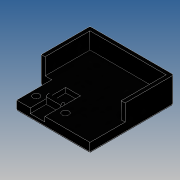
# Autodesk Inventor part: Tapa del cable
Saved by Autodesk Inventor 2016 (Build 200138000, 138)
## iProperties
Created: 2016-05-25
Part Number: Tapa del cable
Material: ABS Plastic
Document SubType Name: Modeling
Designer: Familia
Density: 1.06 g/cm^3
Appearance: Black
Mass: 10.4624 g
Surface Area: 60.6461 cm^2
Volume: 9.87015 cm^3
Author: Familia
Autodesk Inventor part; units mm, degrees
ref_plane "YZ Plane" through (0, 0, 0) normal (1, 0, 0) x (0, 1, 0)
ref_plane "XZ Plane" through (0, 0, 0) normal (0, 1, 0) x (-1, 0, 0)
ref_plane "XY Plane" through (0, 0, 0) normal (0, 0, 1) x (1, 0, 0)
sketch "Sketch1" plane through (0, 0, 0) normal (0, 0, 1) x (1, 0, 0)
  line L0 (-21.5, -21.5) -> (21.5, -21.5)
  line L1 (21.5, -21.5) -> (21.5, 21.5)
  line L2 (21.5, 21.5) -> (-21.5, 21.5)
  line L3 (-21.5, 21.5) -> (-21.5, -21.5)
  line L4 (-21.5, -21.5) -> (21.5, 21.5) construction
  line L5 (21.5, -21.5) -> (-21.5, 21.5) construction
  point P0 (0, 0)
  dimension "d0" = 43
  dimension "d1" = 43
  constraints: 12 end point, 2 midpoint, 2 parallel, 1 horizontal, 1 perpendicular
  measures "d0" distance of L1.end L2.end
  measures "d1" distance of L2.end L0.start
extrude "Extrusion1" add sketch "Sketch1" along normal blind 13.5
sketch "Sketch2" plane through (0, 0, 13.5) normal (0, 0, 1) x (1, 0, 0)
  line L0 (19.5, -19.5) -> (-19.5, -19.5)
  line L1 (-19.5, -19.5) -> (-19.5, 19.5)
  line L2 (-19.5, 19.5) -> (19.5, 19.5)
  line L3 (19.5, 19.5) -> (19.5, -19.5)
  line L4 (19.5, -19.5) -> (-19.5, 19.5) construction
  line L5 (-19.5, -19.5) -> (19.5, 19.5) construction
  line L6 (-21.5, 21.5) -> (-21.5, -21.5) construction
  line L7 (21.5, 21.5) -> (-21.5, 21.5) construction
  point P0 (0, 0)
  dimension "d4" = 2
  dimension "d5" = 2
  constraints: 12 end point, 2 midpoint, 2 parallel, 1 horizontal, 1 perpendicular
  measures "d4" distance between parallel lines of L2 L7
  measures "d5" distance between parallel lines of L6 L1
extrude "Extrusion2" cut sketch "Sketch2" against normal blind 8.5
sketch "Sketch3" plane through (0, 0, 13.5) normal (0, 0, 1) x (1, 0, 0)
  line L0 (-21.5, -3.5) -> (21.5, -3.5)
  line L1 (21.5, -3.5) -> (21.5, -28.5)
  line L2 (21.5, -28.5) -> (-21.5, -28.5)
  line L3 (-21.5, -28.5) -> (-21.5, -3.5)
  line L4 (-21.5, -21.5) -> (21.5, -21.5) projected
  line L5 (-21.5, 21.5) -> (-21.5, -21.5) projected
  line L6 (21.5, -21.5) -> (21.5, 21.5) projected
  point P0 (0, 0)
  dimension "d8" = 18
  dimension "d9" = 25
  constraints: 8 end point, 2 parallel, 2 point on line, 1 horizontal, 1 perpendicular
  measures "d8" distance between parallel lines of L4 L0
  measures "d9" distance between parallel lines of L2 L0
extrude "Extrusion3" cut sketch "Sketch3" against normal up to surface (8.5 mm away)
sketch "Sketch4" plane through (0, 0, 5) normal (0, 0, 1) x (1, 0, 0)
  line L0 (-21.5, -3.5) -> (-19.5, -3.5) projected
  line L1 (21.5, -21.5) -> (-21.5, -21.5) projected
  line L2 (-21.5, -3.5) -> (-16.1, -3.5)
  line L3 (-16.1, -3.5) -> (-16.1, -21.5)
  line L4 (-16.1, -21.5) -> (-21.5, -21.5)
  line L5 (-21.5, -21.5) -> (-21.5, -3.5)
  point P0 (0, 0)
  dimension "d12" = 5.4
  constraints: 8 end point, 2 parallel, 1 horizontal, 1 perpendicular, 1 point on line
  measures "d12" distance between parallel lines of L5 L3
extrude "Extrusion4" cut sketch "Sketch4" against normal through all
sketch "Sketch5" plane through (0, 0, 5) normal (0, 0, 1) x (1, 0, 0)
  line L0 (-9.1, -21.5) -> (-1.6, -21.5)
  line L1 (-1.6, -21.5) -> (-1.6, -3.3)
  line L2 (-1.6, -3.3) -> (-9.1, -3.3)
  line L3 (-9.1, -3.3) -> (-9.1, -21.5)
  line L4 (21.5, -21.5) -> (-16.1, -21.5) construction
  line L5 (-16.1, -3.5) -> (-16.1, -21.5) construction
  line L6 (-12.85, -14.7) -> (-9.1, -14.7) construction
  line L7 (-1.6, -14.7) -> (2.15, -14.7) construction
  point P0 (0, 0)
  dimension "d15" = 7
  dimension "d16" = 7.5
  dimension "d17" = 18.2
  dimension "d18" = 15
  dimension "d19" = 6.8
  constraints: 12 end point, 4 point on line, 2 horizontal, 2 parallel, 2 perpendicular, 1 collinear, 1 horizontal alignment
  measures "d15" distance between parallel lines of L3 L5
  measures "d16" distance of L1.end L2.end
  measures "d17" distance of L0.end L1.end
  measures "d18" distance of L7.end L6.start
  measures "d19" distance from line of L6.start L4
extrude "Extrusion5" cut sketch "Sketch5" against normal blind 2.5
sketch "Sketch6" plane through (0, 0, 2.5) normal (0, 0, 1) x (1, 0, 0)
  line L0 (-9.1, -11.5) -> (-1.6, -11.5)
  line L1 (-1.6, -11.5) -> (-1.6, -13.3)
  line L2 (-1.6, -13.3) -> (-9.1, -13.3)
  line L3 (-9.1, -13.3) -> (-9.1, -11.5)
  line L4 (-9.1, -21.5) -> (-9.1, -3.3) construction
  line L5 (-1.6, -3.3) -> (-1.6, -21.5) construction
  point P0 (0, 0)
  point P1 (-9.1, -12.4)
  dimension "d22" = 1.8
  constraints: 8 end point, 2 midpoint, 2 parallel, 2 point on line, 1 horizontal, 1 perpendicular
  measures "d22" distance between parallel lines of L2 L0
extrude "Extrusion6" add sketch "Sketch6" along normal blind 4.2
full round fillet "Fillet1" first side at (-4.1, -13.3, 3.3333) centre faces at (-6.6, -12.1, 6.7) second side at (-6.6, -11.5, 3.3333)
fillet "Fillet2" radius 0.8 6 edges at (21.5, 21.5, 6.75) (-21.5, 21.5, 6.75) (-21.5, 9, 0) (0, 21.5, 0) (21.5, 0, 0) (2.7, -21.5, 0)
hole "Hole1" at (-12.85, -14.7, 5) at (2.15, -14.7, 5) direction (0, 0, -1) diameter 3.4 end through all clearance for "Flat Head Machine Screw" size "M3" standard "Ansi Metric M Profile"
body "Solid1"
